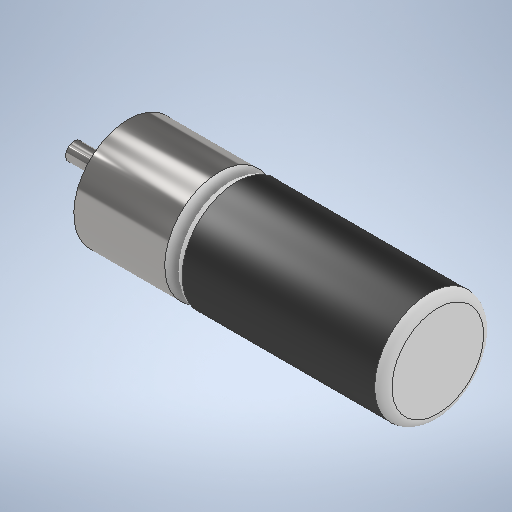
# Autodesk Inventor part: Motor
Saved by Autodesk Inventor 2026 (Build 300175050, 175E)
## iProperties
Created: 2025-08-22
Part Number: Motor
Material: Genérico
Document SubType Name: Modeling
Designer: piero
Density: 1 g/cm^3
Appearance: Valor por defecto
Author: piero
Autodesk Inventor part; units mm, degrees
ref_plane "YZ Plane" through (0, 0, 0) normal (1, 0, 0) x (0, 1, 0)
ref_plane "XZ Plane" through (0, 0, 0) normal (0, 1, 0) x (-1, 0, 0)
ref_plane "XY Plane" through (0, 0, 0) normal (0, 0, 1) x (1, 0, 0)
sketch "Boceto1" plane through (0, 0, 0) normal (0, 0, 1) x (1, 0, 0)
  line L0 (0, 0) -> (10, 0)
  line L1 (10, 0) -> (10, -1.1604)
  line L2 (10, -1.1604) -> (12.5, -1.1604)
  line L3 (12.5, -1.1604) -> (12.5, -9.9104)
  line L4 (12.5, -9.9104) -> (33.5, -9.9104)
  line L5 (35.5, -7.9104) -> (35.5, 12.5896)
  line L6 (33.5, 14.5896) -> (12.5, 14.5896)
  line L7 (12.5, 14.5896) -> (12.5, 5.8396)
  line L8 (12.5, 5.8396) -> (10, 5.8396)
  line L9 (10, 5.8396) -> (10, 4)
  line L10 (10, 4) -> (0, 4)
  line L11 (0, 4) -> (0, 0)
  line L12 (37.5, 14.5896) -> (66.5, 14.5896)
  line L13 (66.5, 14.5896) -> (66.5, -9.9104)
  line L14 (66.5, -9.9104) -> (37.5, -9.9104)
  arc A0 (37.5, 14.5896) -> (35.5, 12.5896) centre (37.5, 12.5896) ccw
  arc A1 (35.5, -7.9104) -> (37.5, -9.9104) centre (37.5, -7.9104) ccw
  arc A2 (35.5, 12.5896) -> (33.5, 14.5896) centre (33.5, 12.5896) ccw
  arc A3 (33.5, -9.9104) -> (35.5, -7.9104) centre (33.5, -7.9104) ccw
  line L15 (66.5, 14.5896) -> (82, 14.5896)
  line L16 (84, 12.5896) -> (84, -7.9104)
  line L17 (82, -9.9104) -> (66.5, -9.9104)
  arc A4 (84, 12.5896) -> (82, 14.5896) centre (82, 12.5896) ccw
  arc A5 (82, -9.9104) -> (84, -7.9104) centre (82, -7.9104) ccw
  line L18 (-5.0848, 2) -> (93.2281, 2)
  point P0 (35.5, -9.9104)
  point P1 (35.5, 14.5896)
  point P2 (11.25, 5.8396)
  point P3 (11.25, -1.1604)
  point P4 (84, 14.5896)
  point P5 (0, 2)
  point P6 (84, 2)
  point P7 (35.5, 12.5896)
  dimension "d0" = 4
  dimension "d1" = 10
  dimension "d2" = 2.5
  dimension "d3" = 7
  dimension "d4" = 24.5
  dimension "d5" = 8.75
  dimension "d6" = 23
  dimension "d7" = 31
  dimension "d8" = 2
  dimension "d9" = 2
  dimension "d10" = 17.5
  dimension "d11" = 2
  dimension "d12" = 2
  constraints: 38 end point, 16 point on line, 12 point on circle, 12 tangent, 11 perpendicular, 6 centre point, 3 equal radius, 2 collinear, 2 horizontal, 2 midpoint
  measures "d0" distance of L0.start L10.end
  measures "d1" distance of L0.start L0.end
  measures "d2" distance of L1.end L2.end
  measures "d3" distance of point (11.25, 5.84) point (11.25, -1.16)
  measures "d4" distance between parallel lines of L6 L4
  measures "d5" distance of L6.end L7.end
  measures "d6" distance of L3.end point (35.5, -9.91)
  measures "d7" distance of point (35.5, 14.59) L12.end
  measures "d8" radius of A0
  measures "d9" radius of A2
  measures "d10" distance of L12.end point (84, 14.59)
  measures "d11" radius of A4
  measures "d12" distance between parallel lines of L0 L18
revolve "Revolución1" add sketch "Boceto1" angle 360 about axis through (-5.0848, 2, 0) along (1, 0, 0) contours L11 L10 L9 L8 L7 L6 A2 L5 L18 | L5 A0 L12 L13 L18 | L13 L15 A4 L16 L18
